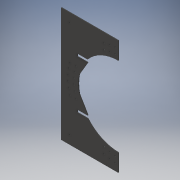
# Autodesk Inventor part: 19in outer coil BOTTOM
Saved by Autodesk Inventor 2016 (Build 200138000, 138)
## iProperties
Created: 2016-01-31
Part Number: 19in outer coil BOTTOM
Material: Copper, Alloy
Document SubType Name: Modeling
Designer: Scott
Density: 8.92 g/cm^3
Appearance: Copper - Satin
Mass: 2218.98 g
Surface Area: 1644.99 cm^2
Volume: 248.765 cm^3
Author: Scott
Autodesk Inventor part; units mm, degrees
ref_plane "YZ Plane" through (0, 0, 0) normal (1, 0, 0) x (0, 1, 0)
ref_plane "XZ Plane" through (0, 0, 0) normal (0, 1, 0) x (-1, 0, 0)
ref_plane "XY Plane" through (0, 0, 0) normal (0, 0, 1) x (1, 0, 0)
sketch "Sketch1" plane through (0, 0, 0) normal (0, 0, 1) x (1, 0, 0)
  circle A0 centre (62.4463, 65.7663) radius 3.175 projected
  circle A1 centre (37.8886, 72.253) radius 3.175 projected
  circle A2 centre (12.7, 75.5236) radius 3.175 projected
  circle A3 centre (12.7, 100.9706) radius 3.175 projected
  circle A4 centre (37.9341, 98.0724) radius 3.175 projected
  circle A5 centre (62.6728, 92.3141) radius 3.175 projected
  circle A6 centre (-62.6728, 92.3141) radius 3.175 projected
  circle A7 centre (-37.9341, 98.0724) radius 3.175 projected
  circle A8 centre (-12.7, 100.9706) radius 3.175 projected
  circle A9 centre (-12.7, 75.5236) radius 3.175 projected
  circle A10 centre (-37.8886, 72.253) radius 3.175 projected
  circle A11 centre (-62.4463, 65.7663) radius 3.175 projected
  circle A12 centre (-196.4399, -108.2163) radius 3.175 projected
  circle A13 centre (-193.1693, -83.0277) radius 3.175 projected
  circle A14 centre (-186.6826, -58.47) radius 3.175 projected
  circle A15 centre (-213.2304, -58.2435) radius 3.175 projected
  circle A16 centre (-218.9887, -82.9822) radius 3.175 projected
  circle A17 centre (-221.8868, -108.2163) radius 3.175 projected
  circle A18 centre (196.4399, -108.2163) radius 3.175 projected
  circle A19 centre (193.1693, -83.0277) radius 3.175 projected
  circle A20 centre (186.6826, -58.47) radius 3.175 projected
  circle A21 centre (213.2304, -58.2435) radius 3.175 projected
  circle A22 centre (218.9887, -82.9822) radius 3.175 projected
  circle A23 centre (221.8868, -108.2163) radius 3.175 projected
  arc A24 (241.3, -120.9163) -> (-241.3, -120.9163) centre (0, -120.9163) ccw projected
  line L0 (-241.3, -120.9163) -> (-177.8, -120.9163) projected
  arc A25 (177.8, -120.9163) -> (-177.8, -120.9163) centre (0, -120.9163) ccw projected
  line L1 (177.8, -120.9163) -> (241.3, -120.9163) projected
  circle A26 centre (-62.4463, -307.5989) radius 3.175 projected
  circle A27 centre (-37.8886, -314.0856) radius 3.175 projected
  circle A28 centre (-12.7, -317.3562) radius 3.175 projected
  circle A29 centre (-12.7, -342.8031) radius 3.175 projected
  circle A30 centre (-37.9341, -339.905) radius 3.175 projected
  circle A31 centre (-62.6728, -334.1466) radius 3.175 projected
  circle A32 centre (62.6728, -334.1466) radius 3.175 projected
  circle A33 centre (37.9341, -339.905) radius 3.175 projected
  circle A34 centre (12.7, -342.8031) radius 3.175 projected
  circle A35 centre (12.7, -317.3562) radius 3.175 projected
  circle A36 centre (37.8886, -314.0856) radius 3.175 projected
  circle A37 centre (62.4463, -307.5989) radius 3.175 projected
  circle A38 centre (196.4399, -133.6163) radius 3.175 projected
  circle A39 centre (193.1693, -158.8048) radius 3.175 projected
  circle A40 centre (186.6826, -183.3626) radius 3.175 projected
  circle A41 centre (213.2304, -183.5891) radius 3.175 projected
  circle A42 centre (218.9887, -158.8504) radius 3.175 projected
  circle A43 centre (221.8868, -133.6163) radius 3.175 projected
  circle A44 centre (-196.4399, -133.6163) radius 3.175 projected
  circle A45 centre (-193.1693, -158.8048) radius 3.175 projected
  circle A46 centre (-186.6826, -183.3626) radius 3.175 projected
  circle A47 centre (-213.2304, -183.5891) radius 3.175 projected
  circle A48 centre (-218.9887, -158.8504) radius 3.175 projected
  circle A49 centre (-221.8868, -133.6163) radius 3.175 projected
  arc A50 (-241.3, -120.9163) -> (241.3, -120.9163) centre (0, -120.9163) ccw projected
  line L2 (241.3, -120.9163) -> (177.8, -120.9163) projected
  arc A51 (-177.8, -120.9163) -> (177.8, -120.9163) centre (0, -120.9163) ccw projected
  line L3 (-177.8, -120.9163) -> (-241.3, -120.9163) projected
  circle A52 centre (0, -120.9163) radius 254
  line L4 (-254, -120.9163) -> (-254, 133.0837)
  line L5 (0, 133.0837) -> (-254, 133.0837)
  line L6 (-254, 100.9706) -> (-254, 104.1456)
  line L7 (-254, 56.8837) -> (-254, 60.0587)
  line L8 (0, -120.9163) -> (-254, 133.0837)
  line L9 (-179.6051, 58.6888) -> (-254, 133.0837)
  circle A53 centre (-216.8026, 95.8863) radius 3.302
  circle A54 centre (259.6856, -120.9163) radius 3.302
  arc A55 (271.0214, -121.5373) -> (259.974, -104.2042) centre (252.2597, -121.3082) ccw
  arc A56 (252.5671, -93.9743) -> (259.974, -104.2042) centre (265.1954, -92.6272) ccw
  line L10 (252.5671, -93.9743) -> (247.0534, -93.9743)
  line L11 (247.0534, -93.9743) -> (247.0534, -120.9163)
  arc A57 (257.0711, -139.4439) -> (271.0214, -121.5373) centre (252.2597, -121.3082) ccw
  arc A58 (257.0711, -139.4439) -> (252.5671, -147.8582) centre (265.1954, -149.2053) ccw
  line L12 (252.5671, -147.8582) -> (247.0534, -147.8582)
  line L13 (247.0534, -147.8582) -> (247.0534, -120.9163)
  line L14 (-254, -120.9163) -> (-254, -374.9163)
  line L15 (-254, -374.9163) -> (0, -374.9163)
  point P0 (0, 0)
  dimension "d0" = 508
  dimension "d3" = 6.604
  dimension "d7" = 6.604
  dimension "d8" = 12.7
  constraints: 24 end point, 12 point on circle, 7 centre point, 3 point on line, 3 tangent, 2 horizontal, 1 coincident, 1 collinear, 1 midpoint, 1 perpendicular, 1 vertical
  measures "d0" diameter of A52
  measures "d3" diameter of A53
  measures "d7" diameter of A54
  measures "d8" radius of A56
extrude "Extrusion1" add sketch "Sketch1" along normal blind 3.175 contours L1 A25 L8 A24 | A50 L0 A51 L1 | L8 A25 L0 A24 | A52 L12 L13 L11 L10 | A52 A56 A55 A57 A58 | L10 L11 L13 L12 A52 | A52 L8 A53 L5 | L15 L14 A52 | A52 L4 L8 A53 | A53 L8 | L8 A53
sketch "Sketch2" plane through (0, 0, 3.175) normal (0, 0, 1) x (1, 0, 0)
  circle A0 centre (259.6856, -120.9163) radius 3.302 projected
  arc A1 (252.5671, -93.9743) -> (0, 133.0837) centre (0, -120.9163) ccw projected
  line L0 (0, 133.0837) -> (-254, 133.0837) projected
  line L1 (-254, 133.0837) -> (-254, -374.9163) projected
  line L2 (-254, -374.9163) -> (0, -374.9163) projected
  arc A2 (0, -374.9163) -> (252.5671, -147.8582) centre (0, -120.9163) ccw projected
  arc A3 (257.0711, -139.4439) -> (252.5671, -147.8582) centre (265.1954, -149.2053) ccw projected
  arc A4 (257.0711, -139.4439) -> (259.974, -104.2042) centre (252.2597, -121.3082) ccw projected
  arc A5 (252.5671, -93.9743) -> (259.974, -104.2042) centre (265.1954, -92.6272) ccw projected
  circle A6 centre (-62.4463, -307.5989) radius 3.175 projected
  circle A7 centre (-37.8886, -314.0856) radius 3.175 projected
  circle A8 centre (-12.7, -317.3562) radius 3.175 projected
  circle A9 centre (-12.7, -342.8031) radius 3.175 projected
  circle A10 centre (-37.9341, -339.905) radius 3.175 projected
  circle A11 centre (-62.6728, -334.1466) radius 3.175 projected
  circle A12 centre (62.6728, -334.1466) radius 3.175 projected
  circle A13 centre (37.9341, -339.905) radius 3.175 projected
  circle A14 centre (12.7, -342.8031) radius 3.175 projected
  circle A15 centre (12.7, -317.3562) radius 3.175 projected
  circle A16 centre (37.8886, -314.0856) radius 3.175 projected
  circle A17 centre (62.4463, -307.5989) radius 3.175 projected
  circle A18 centre (196.4399, -133.6163) radius 3.175 projected
  circle A19 centre (193.1693, -158.8048) radius 3.175 projected
  circle A20 centre (186.6826, -183.3626) radius 3.175 projected
  circle A21 centre (213.2304, -183.5891) radius 3.175 projected
  circle A22 centre (218.9887, -158.8504) radius 3.175 projected
  circle A23 centre (221.8868, -133.6163) radius 3.175 projected
  circle A24 centre (-196.4399, -133.6163) radius 3.175 projected
  circle A25 centre (-193.1693, -158.8048) radius 3.175 projected
  circle A26 centre (-186.6826, -183.3626) radius 3.175 projected
  circle A27 centre (-213.2304, -183.5891) radius 3.175 projected
  circle A28 centre (-218.9887, -158.8504) radius 3.175 projected
  circle A29 centre (-221.8868, -133.6163) radius 3.175 projected
  circle A30 centre (221.8868, -108.2163) radius 3.175 projected
  circle A31 centre (218.9887, -82.9822) radius 3.175 projected
  circle A32 centre (213.2304, -58.2435) radius 3.175 projected
  circle A33 centre (186.6826, -58.47) radius 3.175 projected
  circle A34 centre (193.1693, -83.0277) radius 3.175 projected
  circle A35 centre (196.4399, -108.2163) radius 3.175 projected
  circle A36 centre (-221.8868, -108.2163) radius 3.175 projected
  circle A37 centre (-218.9887, -82.9822) radius 3.175 projected
  circle A38 centre (-213.2304, -58.2435) radius 3.175 projected
  circle A39 centre (-186.6826, -58.47) radius 3.175 projected
  circle A40 centre (-193.1693, -83.0277) radius 3.175 projected
  circle A41 centre (-196.4399, -108.2163) radius 3.175 projected
  circle A42 centre (-62.4463, 65.7663) radius 3.175 projected
  circle A43 centre (-37.8886, 72.253) radius 3.175 projected
  circle A44 centre (-12.7, 75.5236) radius 3.175 projected
  circle A45 centre (-12.7, 100.9706) radius 3.175 projected
  circle A46 centre (-37.9341, 98.0724) radius 3.175 projected
  circle A47 centre (-62.6728, 92.3141) radius 3.175 projected
  circle A48 centre (62.6728, 92.3141) radius 3.175 projected
  circle A49 centre (37.9341, 98.0724) radius 3.175 projected
  circle A50 centre (12.7, 100.9706) radius 3.175 projected
  circle A51 centre (12.7, 75.5236) radius 3.175 projected
  circle A52 centre (37.8886, 72.253) radius 3.175 projected
  circle A53 centre (62.4463, 65.7663) radius 3.175 projected
  circle A54 centre (0, -120.9163) radius 177.8 projected
  line L3 (0, -120.9163) -> (346.8832, -120.9163)
  line L4 (346.8832, -120.9163) -> (346.8832, 148.9285)
  line L5 (346.8832, 148.9285) -> (0, 148.9285)
  line L6 (0, 148.9285) -> (0, -120.9163)
  line L7 (0, -120.9163) -> (432.9103, -120.9163)
  line L8 (432.9103, -120.9163) -> (432.9103, -436.6104)
  line L9 (432.9103, -436.6104) -> (0, -436.6104)
  line L10 (0, -436.6104) -> (0, -120.9163)
  point P0 (0, 0)
  constraints: 16 end point, 4 parallel, 2 horizontal, 2 perpendicular
extrude "Extrusion2" cut sketch "Sketch2" against normal blind 25.4 contours L3 A0 | L3 A4 A3 A2 L10 A54 A0 | A0 L3 | A0 L3 A54 L6 A1 A5 A4 | L3 L7 L8 L9 L10 A2 A3 A4 | A4 A5 A1 L6 L5 L4 L3 | L3 L6 A54 | A54 L10 L3
sketch "Sketch3" plane through (0, 0, 3.175) normal (0, 0, 1) x (1, 0, 0)
  circle A0 centre (-62.6728, 92.3141) radius 3.175 projected
  circle A1 centre (-37.9341, 98.0724) radius 3.175 projected
  circle A2 centre (-12.7, 100.9706) radius 3.175 projected
  circle A3 centre (-12.7, 75.5236) radius 3.175 projected
  circle A4 centre (-37.8886, 72.253) radius 3.175 projected
  circle A5 centre (-62.4463, 65.7663) radius 3.175 projected
  circle A6 centre (-196.4399, -108.2163) radius 3.175 projected
  circle A7 centre (-193.1693, -83.0277) radius 3.175 projected
  circle A8 centre (-186.6826, -58.47) radius 3.175 projected
  circle A9 centre (-213.2304, -58.2435) radius 3.175 projected
  circle A10 centre (-218.9887, -82.9822) radius 3.175 projected
  circle A11 centre (-221.8868, -108.2163) radius 3.175 projected
  circle A12 centre (-221.8868, -133.6163) radius 3.175 projected
  circle A13 centre (-218.9887, -158.8504) radius 3.175 projected
  circle A14 centre (-213.2304, -183.5891) radius 3.175 projected
  circle A15 centre (-186.6826, -183.3626) radius 3.175 projected
  circle A16 centre (-193.1693, -158.8048) radius 3.175 projected
  circle A17 centre (-196.4399, -133.6163) radius 3.175 projected
  circle A18 centre (-62.6728, -334.1466) radius 3.175 projected
  circle A19 centre (-37.9341, -339.905) radius 3.175 projected
  circle A20 centre (-12.7, -342.8031) radius 3.175 projected
  circle A21 centre (-12.7, -317.3562) radius 3.175 projected
  circle A22 centre (-37.8886, -314.0856) radius 3.175 projected
  circle A23 centre (-62.4463, -307.5989) radius 3.175 projected
  line L0 (0, -374.9163) -> (0, -298.7163) projected
  arc A24 (0, 56.8837) -> (0, -298.7163) centre (0, -120.9163) ccw projected
  line L1 (0, 56.8837) -> (0, 133.0837) projected
  line L2 (0, 133.0837) -> (-254, 133.0837) projected
  line L3 (-254, 133.0837) -> (-254, -374.9163) projected
  line L4 (-254, -374.9163) -> (0, -374.9163) projected
  circle A25 centre (-12.7, 100.9706) radius 3.175 projected
  circle A26 centre (-37.9341, 98.0724) radius 3.175 projected
  point P0 (0, 0)
  constraints: 24 coincident
hole "Hole1" at (-12.7, 100.9706, 3.175) at (-12.7, 75.5236, 3.175) at (-37.8886, 72.253, 3.175) at (-37.9341, 98.0724, 3.175) at (-62.6728, 92.3141, 3.175) at (-62.4463, 65.7663, 3.175) at (-186.6826, -58.47, 3.175) at (-213.2304, -58.2435, 3.175) at (-193.1693, -83.0277, 3.175) at (-218.9887, -82.9822, 3.175) at (-196.4399, -108.2163, 3.175) at (-221.8868, -108.2163, 3.175) at (-196.4399, -133.6163, 3.175) at (-221.8868, -133.6163, 3.175) at (-193.1693, -158.8048, 3.175) at (-218.9887, -158.8504, 3.175) at (-213.2304, -183.5891, 3.175) at (-186.6826, -183.3626, 3.175) at (-62.4463, -307.5989, 3.175) at (-62.6728, -334.1466, 3.175) at (-37.9341, -339.905, 3.175) at (-37.8886, -314.0856, 3.175) at (-12.7, -317.3562, 3.175) at (-12.7, -342.8031, 3.175) direction (0, 0, -1) diameter 6.604 end through all
sketch "Sketch4" plane through (0, 0, 3.175) normal (0, 0, 1) x (1, 0, 0)
  circle A0 centre (-12.7, -317.3562) radius 3.302 projected
  circle A1 centre (-37.9341, -339.905) radius 3.302 projected
  circle A2 centre (-62.4463, -307.5989) radius 3.302 projected
  circle A3 centre (-213.2304, -183.5891) radius 3.302 projected
  circle A4 centre (-193.1693, -158.8048) radius 3.302 projected
  circle A5 centre (-196.4399, -133.6163) radius 3.302 projected
  circle A6 centre (-196.4399, -108.2163) radius 3.302 projected
  circle A7 centre (-193.1693, -83.0277) radius 3.302 projected
  circle A8 centre (-186.6826, -58.47) radius 3.302 projected
  circle A9 centre (-62.6728, 92.3141) radius 3.302 projected
  circle A10 centre (-37.8886, 72.253) radius 3.302 projected
  circle A11 centre (-12.7, 100.9706) radius 3.302 projected
  circle A12 centre (-12.7, 75.5236) radius 3.302 projected
  circle A13 centre (-37.9341, 98.0724) radius 3.302 projected
  circle A14 centre (-62.4463, 65.7663) radius 3.302 projected
  circle A15 centre (-213.2304, -58.2435) radius 3.302 projected
  circle A16 centre (-218.9887, -82.9822) radius 3.302 projected
  circle A17 centre (-221.8868, -108.2163) radius 3.302 projected
  circle A18 centre (-221.8868, -133.6163) radius 3.302 projected
  circle A19 centre (-218.9887, -158.8504) radius 3.302 projected
  circle A20 centre (-186.6826, -183.3626) radius 3.302 projected
  circle A21 centre (-62.6728, -334.1466) radius 3.302 projected
  circle A22 centre (-37.8886, -314.0856) radius 3.302 projected
  circle A23 centre (-12.7, -342.8031) radius 3.302 projected
  line L0 (0, -374.9163) -> (0, -298.7163) projected
  arc A24 (0, 56.8837) -> (0, -298.7163) centre (0, -120.9163) ccw projected
  line L1 (0, 56.8837) -> (0, 133.0837) projected
  line L2 (0, 133.0837) -> (-254, 133.0837) projected
  line L3 (-254, 133.0837) -> (-254, -374.9163) projected
  line L4 (-254, -374.9163) -> (0, -374.9163) projected
  line L5 (-254, 133.0837) -> (0, -120.9163)
  line L6 (-254, 133.0837) -> (-254, -374.9163) projected
  line L7 (0, -120.9163) -> (-254, -374.9163)
  circle A25 centre (-215.9, 94.9837) radius 3.302
  circle A26 centre (-215.9, -336.8163) radius 3.302
  point P0 (0, 0)
  dimension "d20" = 6.604
  dimension "d21" = 6.604
  dimension "d22" = 38.1
  dimension "d23" = 38.1
  constraints: 4 end point, 2 centre point, 2 point on line, 1 perpendicular
  measures "d20" diameter of A26
  measures "d21" diameter of A25
  measures "d22" horizontal distance of L2.end A25.centre
  measures "d23" distance from line of L3 A26.centre
extrude "Extrusion3" cut sketch "Sketch4" against normal blind 25.4 contours A26 L7 | L7 A26 | A25 L5 | L5 A25
sketch "Sketch5" plane through (0, 0, 3.175) normal (0, 0, 1) x (1, 0, 0)
  line L0 (0, 0) -> (0, -62.5604)
  line L1 (183.162, -19.3163) -> (145.9119, -19.3163) projected
  arc A0 (145.9119, -222.5163) -> (145.9119, -19.3163) centre (0, -120.9163) ccw projected
  line L2 (145.9119, -222.5163) -> (183.162, -222.5163) projected
  line L3 (183.162, -222.5163) -> (183.162, -235.2163) projected
  line L4 (183.162, -235.2163) -> (136.1923, -235.2163) projected
  arc A1 (0, -298.7163) -> (136.1923, -235.2163) centre (0, -120.9163) ccw projected
  line L5 (0, -298.7163) -> (0, -374.9163) projected
  arc A2 (0, -374.9163) -> (249.0244, -170.945) centre (0, -120.9163) ccw projected
  arc A3 (256.4729, -157.4946) -> (249.0244, -170.945) centre (273.9268, -175.9478) ccw projected
  arc A4 (256.4729, -157.4946) -> (256.4729, -84.338) centre (221.8757, -120.9163) ccw projected
  arc A5 (249.0244, -70.8876) -> (256.4729, -84.338) centre (273.9268, -65.8847) ccw projected
  arc A6 (249.0244, -70.8876) -> (0, 133.0837) centre (0, -120.9163) ccw projected
  line L6 (0, 133.0837) -> (0, 56.8837) projected
  arc A7 (136.1923, -6.6163) -> (0, 56.8837) centre (0, -120.9163) ccw projected
  line L7 (136.1923, -6.6163) -> (183.162, -6.6163) projected
  line L8 (183.162, -6.6163) -> (183.162, -19.3163) projected
  circle A8 centre (12.7, 75.5236) radius 3.302 projected
  circle A9 centre (37.9341, 98.0724) radius 3.302 projected
  circle A10 centre (62.4463, 65.7663) radius 3.302 projected
  circle A11 centre (186.6826, -58.47) radius 3.302 projected
  circle A12 centre (218.9887, -82.9822) radius 3.302 projected
  circle A13 centre (196.4399, -108.2163) radius 3.302 projected
  circle A14 centre (221.8868, -133.6163) radius 3.302 projected
  circle A15 centre (193.1693, -158.8048) radius 3.302 projected
  circle A16 centre (213.2304, -183.5891) radius 3.302 projected
  circle A17 centre (12.7, -317.3562) radius 3.302 projected
  circle A18 centre (37.8886, -314.0856) radius 3.302 projected
  circle A19 centre (62.4463, -307.5989) radius 3.302 projected
  circle A20 centre (62.6728, -334.1466) radius 3.302 projected
  circle A21 centre (37.9341, -339.905) radius 3.302 projected
  circle A22 centre (12.7, -342.8031) radius 3.302 projected
  circle A23 centre (186.6826, -183.3626) radius 3.302 projected
  circle A24 centre (218.9887, -158.8504) radius 3.302 projected
  circle A25 centre (196.4399, -133.6163) radius 3.302 projected
  circle A26 centre (221.8868, -108.2163) radius 3.302 projected
  circle A27 centre (193.1693, -83.0277) radius 3.302 projected
  circle A28 centre (213.2304, -58.2435) radius 3.302 projected
  circle A29 centre (62.6728, 92.3141) radius 3.302 projected
  circle A30 centre (37.8886, 72.253) radius 3.302 projected
  circle A31 centre (12.7, 100.9706) radius 3.302 projected
  circle A32 centre (259.6856, -120.9163) radius 3.302 projected
  line L9 (183.162, -6.6163) -> (93.7815, -6.6163)
  line L10 (93.7815, -6.6163) -> (93.7815, -19.3163)
  line L11 (93.7815, -19.3163) -> (183.162, -19.3163)
  line L12 (183.162, -19.3163) -> (183.162, -6.6163)
  line L13 (183.162, -222.5163) -> (79.4592, -222.5163)
  line L14 (79.4592, -222.5163) -> (79.4592, -235.2163)
  line L15 (79.4592, -235.2163) -> (183.162, -235.2163)
  line L16 (183.162, -235.2163) -> (183.162, -222.5163)
  line L17 (-183.162, -222.5163) -> (-183.162, -235.2163)
  line L18 (-136.1923, -6.6163) -> (-183.162, -6.6163)
  line L19 (-183.162, -6.6163) -> (-183.162, -19.3163)
  line L20 (-93.7815, -6.6163) -> (-93.7815, -19.3163)
  line L21 (-93.7815, -19.3163) -> (-183.162, -19.3163)
  line L22 (-183.162, -222.5163) -> (-79.4592, -222.5163)
  line L23 (-79.4592, -222.5163) -> (-79.4592, -235.2163)
  line L24 (-79.4592, -235.2163) -> (-183.162, -235.2163)
  line L25 (-183.162, -6.6163) -> (-93.7815, -6.6163)
  line L26 (-93.7815, -6.6163) -> (-93.7815, -19.3163)
  line L27 (-93.7815, -19.3163) -> (-183.162, -19.3163)
  line L28 (-183.162, -19.3163) -> (-183.162, -6.6163)
  line L29 (-183.162, -222.5163) -> (-79.4592, -222.5163)
  line L30 (-79.4592, -222.5163) -> (-79.4592, -235.2163)
  line L31 (-79.4592, -235.2163) -> (-183.162, -235.2163)
  line L32 (-183.162, -235.2163) -> (-183.162, -222.5163)
  constraints: 44 end point, 11 symmetric about line, 8 parallel, 4 horizontal, 4 perpendicular, 1 vertical
extrude "Extrusion4" cut sketch "Sketch5" against normal blind 25.4 contours L22 L23 L24 L17 | L25 L20 L21 L19 L18
sketch "Sketch6" plane through (0, 0, 3.175) normal (0, 0, 1) x (1, 0, 0)
  line L0 (-145.9119, -19.3163) -> (-183.162, -19.3163) projected
  line L1 (-183.162, -19.3163) -> (-183.162, -6.6163) projected
  line L2 (-183.162, -6.6163) -> (-136.1923, -6.6163) projected
  arc A0 (0, 56.8837) -> (-136.1923, -6.6163) centre (0, -120.9163) ccw projected
  line L3 (0, 56.8837) -> (0, 133.0837) projected
  line L4 (0, 133.0837) -> (-254, 133.0837) projected
  line L5 (-254, 133.0837) -> (-254, -374.9163) projected
  line L6 (-254, -374.9163) -> (0, -374.9163) projected
  line L7 (0, -374.9163) -> (0, -298.7163) projected
  arc A1 (-136.1923, -235.2163) -> (0, -298.7163) centre (0, -120.9163) ccw projected
  line L8 (-136.1923, -235.2163) -> (-183.162, -235.2163) projected
  line L9 (-183.162, -235.2163) -> (-183.162, -222.5163) projected
  line L10 (-183.162, -222.5163) -> (-145.9119, -222.5163) projected
  arc A2 (-145.9119, -19.3163) -> (-145.9119, -222.5163) centre (0, -120.9163) ccw projected
  circle A3 centre (-12.7, -342.8031) radius 3.302 projected
  circle A4 centre (-37.8886, -314.0856) radius 3.302 projected
  circle A5 centre (-62.6728, -334.1466) radius 3.302 projected
  circle A6 centre (-186.6826, -183.3626) radius 3.302 projected
  circle A7 centre (-218.9887, -158.8504) radius 3.302 projected
  circle A8 centre (-221.8868, -133.6163) radius 3.302 projected
  circle A9 centre (-221.8868, -108.2163) radius 3.302 projected
  circle A10 centre (-218.9887, -82.9822) radius 3.302 projected
  circle A11 centre (-213.2304, -58.2435) radius 3.302 projected
  circle A12 centre (-62.4463, 65.7663) radius 3.302 projected
  circle A13 centre (-37.9341, 98.0724) radius 3.302 projected
  circle A14 centre (-12.7, 75.5236) radius 3.302 projected
  circle A15 centre (-12.7, 100.9706) radius 3.302 projected
  circle A16 centre (-37.8886, 72.253) radius 3.302 projected
  circle A17 centre (-62.6728, 92.3141) radius 3.302 projected
  circle A18 centre (-186.6826, -58.47) radius 3.302 projected
  circle A19 centre (-193.1693, -83.0277) radius 3.302 projected
  circle A20 centre (-196.4399, -108.2163) radius 3.302 projected
  circle A21 centre (-196.4399, -133.6163) radius 3.302 projected
  circle A22 centre (-193.1693, -158.8048) radius 3.302 projected
  circle A23 centre (-213.2304, -183.5891) radius 3.302 projected
  circle A24 centre (-62.4463, -307.5989) radius 3.302 projected
  circle A25 centre (-37.9341, -339.905) radius 3.302 projected
  circle A26 centre (-12.7, -317.3562) radius 3.302 projected
  circle A27 centre (-215.9, 94.9837) radius 3.302 projected
  circle A28 centre (-215.9, -336.8163) radius 3.302 projected
  line L11 (183.162, -19.3163) -> (136.1923, -19.3163) projected
  line L12 (136.1923, -19.3163) -> (173.6699, -82.8163) projected
  arc A29 (177.8, -120.9163) -> (173.6699, -82.8163) centre (0, -120.9163) ccw projected
  line L13 (177.8, -120.9163) -> (241.3, -120.9163) projected
  arc A30 (241.3, -120.9163) -> (-241.3, -120.9163) centre (0, -120.9163) ccw projected
  line L14 (-241.3, -120.9163) -> (-177.8, -120.9163) projected
  arc A31 (-173.6699, -82.8163) -> (-177.8, -120.9163) centre (0, -120.9163) ccw projected
  line L15 (-173.6699, -82.8163) -> (-136.1923, -19.3163) projected
  line L16 (-136.1923, -19.3163) -> (-183.162, -19.3163) projected
  line L17 (-183.162, -19.3163) -> (-183.162, -6.6163) projected
  line L18 (-183.162, -6.6163) -> (-136.1923, -6.6163) projected
  arc A32 (136.1923, -6.6163) -> (-136.1923, -6.6163) centre (0, -120.9163) ccw projected
  line L19 (136.1923, -6.6163) -> (183.162, -6.6163) projected
  line L20 (183.162, -6.6163) -> (183.162, -19.3163) projected
  circle A33 centre (62.4463, 65.7663) radius 3.175 projected
  circle A34 centre (37.8886, 72.253) radius 3.175 projected
  circle A35 centre (12.7, 75.5236) radius 3.175 projected
  circle A36 centre (12.7, 100.9706) radius 3.175 projected
  circle A37 centre (37.9341, 98.0724) radius 3.175 projected
  circle A38 centre (62.6728, 92.3141) radius 3.175 projected
  circle A39 centre (-62.6728, 92.3141) radius 3.175 projected
  circle A40 centre (-37.9341, 98.0724) radius 3.175 projected
  circle A41 centre (-12.7, 100.9706) radius 3.175 projected
  circle A42 centre (-12.7, 75.5236) radius 3.175 projected
  circle A43 centre (-37.8886, 72.253) radius 3.175 projected
  circle A44 centre (-62.4463, 65.7663) radius 3.175 projected
  circle A45 centre (-196.4399, -108.2163) radius 3.175 projected
  circle A46 centre (-193.1693, -83.0277) radius 3.175 projected
  circle A47 centre (-186.6826, -58.47) radius 3.175 projected
  circle A48 centre (-213.2304, -58.2435) radius 3.175 projected
  circle A49 centre (-218.9887, -82.9822) radius 3.175 projected
  circle A50 centre (-221.8868, -108.2163) radius 3.175 projected
  circle A51 centre (196.4399, -108.2163) radius 3.175 projected
  circle A52 centre (193.1693, -83.0277) radius 3.175 projected
  circle A53 centre (186.6826, -58.47) radius 3.175 projected
  circle A54 centre (213.2304, -58.2435) radius 3.175 projected
  circle A55 centre (218.9887, -82.9822) radius 3.175 projected
  circle A56 centre (221.8868, -108.2163) radius 3.175 projected
  line L21 (-183.162, -222.5163) -> (-136.1923, -222.5163) projected
  line L22 (-136.1923, -222.5163) -> (-173.6699, -159.0163) projected
  arc A57 (-177.8, -120.9163) -> (-173.6699, -159.0163) centre (0, -120.9163) ccw projected
  line L23 (-177.8, -120.9163) -> (-241.3, -120.9163) projected
  arc A58 (-241.3, -120.9163) -> (241.3, -120.9163) centre (0, -120.9163) ccw projected
  line L24 (241.3, -120.9163) -> (177.8, -120.9163) projected
  arc A59 (173.6699, -159.0163) -> (177.8, -120.9163) centre (0, -120.9163) ccw projected
  line L25 (173.6699, -159.0163) -> (136.1923, -222.5163) projected
  line L26 (136.1923, -222.5163) -> (183.162, -222.5163) projected
  line L27 (183.162, -222.5163) -> (183.162, -235.2163) projected
  line L28 (183.162, -235.2163) -> (136.1923, -235.2163) projected
  arc A60 (-136.1923, -235.2163) -> (136.1923, -235.2163) centre (0, -120.9163) ccw projected
  line L29 (-136.1923, -235.2163) -> (-183.162, -235.2163) projected
  line L30 (-183.162, -235.2163) -> (-183.162, -222.5163) projected
  circle A61 centre (-62.4463, -307.5989) radius 3.175 projected
  circle A62 centre (-37.8886, -314.0856) radius 3.175 projected
  circle A63 centre (-12.7, -317.3562) radius 3.175 projected
  circle A64 centre (-12.7, -342.8031) radius 3.175 projected
  circle A65 centre (-37.9341, -339.905) radius 3.175 projected
  circle A66 centre (-62.6728, -334.1466) radius 3.175 projected
  circle A67 centre (62.6728, -334.1466) radius 3.175 projected
  circle A68 centre (37.9341, -339.905) radius 3.175 projected
  circle A69 centre (12.7, -342.8031) radius 3.175 projected
  circle A70 centre (12.7, -317.3562) radius 3.175 projected
  circle A71 centre (37.8886, -314.0856) radius 3.175 projected
  circle A72 centre (62.4463, -307.5989) radius 3.175 projected
  circle A73 centre (196.4399, -133.6163) radius 3.175 projected
  circle A74 centre (193.1693, -158.8048) radius 3.175 projected
  circle A75 centre (186.6826, -183.3626) radius 3.175 projected
  circle A76 centre (213.2304, -183.5891) radius 3.175 projected
  circle A77 centre (218.9887, -158.8504) radius 3.175 projected
  circle A78 centre (221.8868, -133.6163) radius 3.175 projected
  circle A79 centre (-196.4399, -133.6163) radius 3.175 projected
  circle A80 centre (-193.1693, -158.8048) radius 3.175 projected
  circle A81 centre (-186.6826, -183.3626) radius 3.175 projected
  circle A82 centre (-213.2304, -183.5891) radius 3.175 projected
  circle A83 centre (-218.9887, -158.8504) radius 3.175 projected
  circle A84 centre (-221.8868, -133.6163) radius 3.175 projected
  arc A85 (-145.9119, -19.3163) -> (-145.9119, -222.5163) centre (0, -120.9163) ccw projected
  arc A86 (-173.6699, -159.0163) -> (-145.9119, -19.3163) centre (0, -120.9163) ccw
  line L31 (-173.6699, -159.0163) -> (-136.1923, -222.5163)
  line L32 (-183.162, -222.5163) -> (-145.9119, -222.5163) projected
  line L33 (-136.1923, -222.5163) -> (-145.9119, -222.5163)
  point P0 (0, 0)
  constraints: 4 end point, 2 point on circle, 1 centre point, 1 collinear
extrude "Extrusion5" add sketch "Sketch6" against normal blind 3.175 contours L16 L15 A2 | L22 L21 A2
body "Solid1"
